Autodesk Inventor part; units mm, degrees
(part 2 of 3)
  line L709 (86.8713, 6.9678) -> (87.2019, 6.7467) construction
  line L710 (87.2019, 6.7467) -> (87.5411, 6.5326) construction
  line L711 (87.5411, 6.5326) -> (87.8883, 6.3253) construction
  line L712 (87.8883, 6.3253) -> (88.2432, 6.1246) construction
  line L713 (88.2432, 6.1246) -> (88.6055, 5.9303) construction
  line L714 (88.6055, 5.9303) -> (88.9749, 5.7423) construction
  line L715 (88.9749, 5.7423) -> (89.3511, 5.5606) construction
  line L716 (89.3511, 5.5606) -> (89.7339, 5.3851) construction
  line L717 (89.7339, 5.3851) -> (90.1231, 5.2157) construction
  line L718 (90.1231, 5.2157) -> (90.5185, 5.0524) construction
  line L719 (90.5185, 5.0524) -> (90.92, 4.8952) construction
  line L720 (90.92, 4.8952) -> (91.3274, 4.7441) construction
  line L721 (91.3274, 4.7441) -> (91.7405, 4.599) construction
  line L722 (91.7405, 4.599) -> (92.1592, 4.46) construction
  line L723 (92.1592, 4.46) -> (92.4356, 4.6954) construction
  line L724 (92.4356, 4.6954) -> (92.7102, 4.9328) construction
  line L725 (92.7102, 4.9328) -> (92.9832, 5.1722) construction
  line L726 (92.9832, 5.1722) -> (93.2544, 5.4136) construction
  line L727 (93.2544, 5.4136) -> (93.5238, 5.657) construction
  line L728 (93.5238, 5.657) -> (93.7914, 5.9023) construction
  line L729 (93.7914, 5.9023) -> (94.0572, 6.1495) construction
  line L730 (94.0572, 6.1495) -> (94.3213, 6.3987) construction
  line L731 (94.3213, 6.3987) -> (94.5835, 6.6498) construction
  line L732 (94.5835, 6.6498) -> (94.8439, 6.9028) construction
  line L733 (94.8439, 6.9028) -> (94.7449, 7.3328) construction
  line L734 (94.7449, 7.3328) -> (94.6393, 7.7577) construction
  line L735 (94.6393, 7.7577) -> (94.5272, 8.1775) construction
  line L736 (94.5272, 8.1775) -> (94.4085, 8.592) construction
  line L737 (94.4085, 8.592) -> (94.2832, 9.001) construction
  line L738 (94.2832, 9.001) -> (94.1512, 9.4044) construction
  line L739 (94.1512, 9.4044) -> (94.0125, 9.8021) construction
  line L740 (94.0125, 9.8021) -> (93.867, 10.1937) construction
  line L741 (93.867, 10.1937) -> (93.7146, 10.5791) construction
  line L742 (93.7146, 10.5791) -> (93.5553, 10.9581) construction
  line L743 (93.5553, 10.9581) -> (93.3889, 11.3303) construction
  line L744 (93.3889, 11.3303) -> (93.2152, 11.6955) construction
  line L745 (93.2152, 11.6955) -> (93.034, 12.0533) construction
  line L746 (93.034, 12.0533) -> (92.845, 12.4033) construction
  line L747 (92.845, 12.4033) -> (92.6478, 12.7449) construction
  line L748 (92.6478, 12.7449) -> (92.442, 13.0774) construction
  line L749 (92.442, 13.0774) -> (92.2268, 13.3998) construction
  line L750 (92.2268, 13.3998) -> (92.001, 13.7108) construction
  line L751 (92.001, 13.7108) -> (91.7626, 14.008) construction
  line L752 (91.7626, 14.008) -> (91.5055, 14.2844) construction
  line L753 (91.5055, 14.2844) -> (91.4052, 14.3817) construction
  line L754 (91.4052, 14.3817) -> (88.6168, 16.8782) construction
  arc A46 (88.1374, 17.5249) -> (88.6168, 16.8782) centre (89.9509, 18.3683) ccw construction
  line L755 (88.1374, 17.5249) -> (73.8914, 48.1593) construction
  line L756 (73.8914, 48.1593) -> (60.7972, 80.3007) construction
  arc A47 (60.6816, 80.6977) -> (60.7972, 80.3007) centre (62.6494, 81.0553) ccw construction
  line L757 (60.6816, 80.6977) -> (53.4682, 120.3931) construction
  circle A48 centre (-1.8122, 42.5) radius 4 construction
  line L758 (-3.103, 31.8278) -> (-3.0572, 31.8223) construction
  line L759 (-3.0572, 31.8223) -> (-3.0114, 31.8171) construction
  line L760 (-3.0114, 31.8171) -> (-2.9655, 31.8121) construction
  line L761 (-2.9655, 31.8121) -> (-2.9197, 31.8072) construction
  line L762 (-2.9197, 31.8072) -> (-2.8738, 31.8026) construction
  line L763 (-2.8738, 31.8026) -> (-2.5758, 31.7487) construction
  line L764 (-2.5758, 31.7487) -> (-2.3607, 31.6779) construction
  line L765 (-2.3607, 31.6779) -> (-2.1282, 31.5901) construction
  line L766 (-2.1282, 31.5901) -> (-1.9375, 31.49) construction
  line L767 (-1.9375, 31.49) -> (-1.7706, 31.3775) construction
  line L768 (-1.7706, 31.3775) -> (-1.6217, 31.2529) construction
  line L769 (-1.6217, 31.2529) -> (-1.477, 31.1167) construction
  line L770 (-1.477, 31.1167) -> (-1.3373, 30.9695) construction
  line L771 (-1.3373, 30.9695) -> (-1.2159, 30.8111) construction
  line L772 (-1.2159, 30.8111) -> (-1.1122, 30.6413) construction
  line L773 (-1.1122, 30.6413) -> (-1.013, 30.4611) construction
  line L774 (-1.013, 30.4611) -> (-0.9213, 30.2706) construction
  line L775 (-0.9213, 30.2706) -> (-0.8507, 30.0687) construction
  line L776 (-0.8507, 30.0687) -> (-0.7921, 29.8564) construction
  line L777 (-0.7921, 29.8564) -> (-0.7363, 29.6344) construction
  line L778 (-0.7363, 29.6344) -> (-0.7072, 29.401) construction
  line L779 (-0.7072, 29.401) -> (-0.6823, 29.1582) construction
  line L780 (-0.6823, 29.1582) -> (-0.6727, 28.9053) construction
  line L781 (-0.6727, 28.9053) -> (-0.6907, 28.6416) construction
  line L782 (-0.6907, 28.6416) -> (-0.701, 28.3702) construction
  line L783 (-0.701, 28.3702) -> (-0.5986, 27.9953) construction
  line L784 (-0.5986, 27.9953) -> (-0.4487, 27.625) construction
  line L785 (-0.4487, 27.625) -> (-0.2641, 27.2592) construction
  line L786 (-0.2641, 27.2592) -> (-0.0491, 26.8981) construction
  line L787 (-0.0491, 26.8981) -> (0.1935, 26.5424) construction
  line L788 (0.1935, 26.5424) -> (0.4621, 26.1928) construction
  line L789 (0.4621, 26.1928) -> (0.7554, 25.8498) construction
  line L790 (0.7554, 25.8498) -> (1.0724, 25.5143) construction
  line L791 (1.0724, 25.5143) -> (1.4124, 25.1869) construction
  line L792 (1.4124, 25.1869) -> (1.7746, 24.8683) construction
  line L793 (1.7746, 24.8683) -> (2.1584, 24.5594) construction
  line L794 (2.1584, 24.5594) -> (2.5632, 24.2608) construction
  line L795 (2.5632, 24.2608) -> (2.9885, 23.9733) construction
  line L796 (2.9885, 23.9733) -> (3.4338, 23.6976) construction
  line L797 (3.4338, 23.6976) -> (3.8985, 23.4344) construction
  line L798 (3.8985, 23.4344) -> (4.3822, 23.1845) construction
  line L799 (4.3822, 23.1845) -> (4.8844, 22.9487) construction
  line L800 (4.8844, 22.9487) -> (5.4044, 22.7275) construction
  line L801 (5.4044, 22.7275) -> (5.9419, 22.5218) construction
  line L802 (5.9419, 22.5218) -> (6.4962, 22.3322) construction
  line L803 (6.4962, 22.3322) -> (6.5464, 22.3529) construction
  line L804 (6.5464, 22.3529) -> (6.5966, 22.3738) construction
  line L805 (6.5966, 22.3738) -> (6.6467, 22.3948) construction
  line L806 (6.6467, 22.3948) -> (6.6967, 22.4159) construction
  line L807 (6.6967, 22.4159) -> (6.7467, 22.4372) construction
  line L808 (6.7467, 22.4372) -> (6.7967, 22.4586) construction
  line L809 (6.7967, 22.4586) -> (6.8466, 22.4801) construction
  line L810 (6.8466, 22.4801) -> (6.8964, 22.5017) construction
  line L811 (6.8964, 22.5017) -> (6.9462, 22.5235) construction
  line L812 (6.9462, 22.5235) -> (6.996, 22.5454) construction
  line L813 (6.996, 22.5454) -> (7.2427, 23.0767) construction
  line L814 (7.2427, 23.0767) -> (7.4661, 23.607) construction
  line L815 (7.4661, 23.607) -> (7.6664, 24.1355) construction
  line L816 (7.6664, 24.1355) -> (7.8437, 24.6612) construction
  line L817 (7.8437, 24.6612) -> (7.998, 25.1833) construction
  line L818 (7.998, 25.1833) -> (8.1297, 25.7009) construction
  line L819 (8.1297, 25.7009) -> (8.2389, 26.2131) construction
  line L820 (8.2389, 26.2131) -> (8.3257, 26.7191) construction
  line L821 (8.3257, 26.7191) -> (8.3903, 27.218) construction
  line L822 (8.3903, 27.218) -> (8.4329, 27.7088) construction
  line L823 (8.4329, 27.7088) -> (8.4536, 28.1907) construction
  line L824 (8.4536, 28.1907) -> (8.4525, 28.6627) construction
  line L825 (8.4525, 28.6627) -> (8.4297, 29.1237) construction
  line L826 (8.4297, 29.1237) -> (8.3851, 29.5728) construction
  line L827 (8.3851, 29.5728) -> (8.3186, 30.0087) construction
  line L828 (8.3186, 30.0087) -> (8.2298, 30.43) construction
  line L829 (8.2298, 30.43) -> (8.1179, 30.835) construction
  line L830 (8.1179, 30.835) -> (7.9816, 31.2215) construction
  line L831 (7.9816, 31.2215) -> (7.818, 31.5859) construction
  line L832 (7.818, 31.5859) -> (7.6183, 31.9192) construction
  line L833 (7.6183, 31.9192) -> (7.4153, 32.0996) construction
  line L834 (7.4153, 32.0996) -> (7.2125, 32.2692) construction
  line L835 (7.2125, 32.2692) -> (7.0366, 32.4511) construction
  line L836 (7.0366, 32.4511) -> (6.8786, 32.6371) construction
  line L837 (6.8786, 32.6371) -> (6.7302, 32.8196) construction
  line L838 (6.7302, 32.8196) -> (6.6086, 33.0136) construction
  line L839 (6.6086, 33.0136) -> (6.4959, 33.2028) construction
  line L840 (6.4959, 33.2028) -> (6.399, 33.3935) construction
  line L841 (6.399, 33.3935) -> (6.3249, 33.5916) construction
  line L842 (6.3249, 33.5916) -> (6.2635, 33.7878) construction
  line L843 (6.2635, 33.7878) -> (6.2127, 33.9802) construction
  line L844 (6.2127, 33.9802) -> (6.1824, 34.1775) construction
  line L845 (6.1824, 34.1775) -> (6.1728, 34.3802) construction
  line L846 (6.1728, 34.3802) -> (6.1746, 34.5788) construction
  line L847 (6.1746, 34.5788) -> (6.1877, 34.7726) construction
  line L848 (6.1877, 34.7726) -> (6.2221, 34.971) construction
  line L849 (6.2221, 34.971) -> (6.2818, 35.1778) construction
  line L850 (6.2818, 35.1778) -> (6.3793, 35.4064) construction
  line L851 (6.3793, 35.4064) -> (6.477, 35.6107) construction
  line L852 (6.477, 35.6107) -> (6.6444, 35.8631) construction
  line L853 (6.6444, 35.8631) -> (6.6728, 35.8994) construction
  line L854 (6.6728, 35.8994) -> (6.701, 35.9359) construction
  line L855 (6.701, 35.9359) -> (6.7291, 35.9725) construction
  line L856 (6.7291, 35.9725) -> (6.7571, 36.0092) construction
  line L857 (6.7571, 36.0092) -> (6.7848, 36.046) construction
  line L858 (6.7848, 36.046) -> (6.8124, 36.0829) construction
  line L859 (6.8124, 36.0829) -> (6.8399, 36.12) construction
  line L860 (6.8399, 36.12) -> (6.8672, 36.1572) construction
  line L861 (6.8672, 36.1572) -> (6.8943, 36.1945) construction
  line L862 (6.8943, 36.1945) -> (6.9213, 36.2319) construction
  line L863 (6.9213, 36.2319) -> (7.1169, 36.4631) construction
  line L864 (7.1169, 36.4631) -> (7.2858, 36.6139) construction
  line L865 (7.2858, 36.6139) -> (7.4781, 36.7713) construction
  line L866 (7.4781, 36.7713) -> (7.6601, 36.8864) construction
  line L867 (7.6601, 36.8864) -> (7.841, 36.9748) construction
  line L868 (7.841, 36.9748) -> (8.0234, 37.0414) construction
  line L869 (8.0234, 37.0414) -> (8.2136, 37.0986) construction
  line L870 (8.2136, 37.0986) -> (8.4109, 37.146) construction
  line L871 (8.4109, 37.146) -> (8.6089, 37.1719) construction
  line L872 (8.6089, 37.1719) -> (8.8077, 37.1769) construction
  line L873 (8.8077, 37.1769) -> (9.0134, 37.1726) construction
  line L874 (9.0134, 37.1726) -> (9.2243, 37.1568) construction
  line L875 (9.2243, 37.1568) -> (9.4344, 37.117) construction
  line L876 (9.4344, 37.117) -> (9.6476, 37.0616) construction
  line L877 (9.6476, 37.0616) -> (9.8677, 36.9989) construction
  line L878 (9.8677, 36.9989) -> (10.0844, 36.9074) construction
  line L879 (10.0844, 36.9074) -> (10.3071, 36.8076) construction
  line L880 (10.3071, 36.8076) -> (10.5309, 36.6895) construction
  line L881 (10.5309, 36.6895) -> (10.7503, 36.5421) construction
  line L882 (10.7503, 36.5421) -> (10.9802, 36.3974) construction
  line L883 (10.9802, 36.3974) -> (11.3561, 36.2987) construction
  line L884 (11.3561, 36.2987) -> (11.7516, 36.2433) construction
  line L885 (11.7516, 36.2433) -> (12.1608, 36.2203) construction
  line L886 (12.1608, 36.2203) -> (12.581, 36.2259) construction
  line L887 (12.581, 36.2259) -> (13.0103, 36.2582) construction
  line L888 (13.0103, 36.2582) -> (13.4474, 36.316) construction
  line L889 (13.4474, 36.316) -> (13.8911, 36.3985) construction
  line L890 (13.8911, 36.3985) -> (14.3402, 36.5053) construction
  line L891 (14.3402, 36.5053) -> (14.7937, 36.636) construction
  line L892 (14.7937, 36.636) -> (15.2507, 36.7904) construction
  line L893 (15.2507, 36.7904) -> (15.7101, 36.9683) construction
  line L894 (15.7101, 36.9683) -> (16.1711, 37.1696) construction
  line L895 (16.1711, 37.1696) -> (16.6328, 37.3941) construction
  line L896 (16.6328, 37.3941) -> (17.0942, 37.6419) construction
  line L897 (17.0942, 37.6419) -> (17.5545, 37.9128) construction
  line L898 (17.5545, 37.9128) -> (18.0127, 38.2068) construction
  line L899 (18.0127, 38.2068) -> (18.4681, 38.5237) construction
  line L900 (18.4681, 38.5237) -> (18.9196, 38.8635) construction
  line L901 (18.9196, 38.8635) -> (19.3665, 39.2261) construction
  line L902 (19.3665, 39.2261) -> (19.8079, 39.6113) construction
  line L903 (19.8079, 39.6113) -> (19.815, 39.6652) construction
  line L904 (19.815, 39.6652) -> (19.822, 39.7191) construction
  line L905 (19.822, 39.7191) -> (19.8289, 39.773) construction
  line L906 (19.8289, 39.773) -> (19.8356, 39.8269) construction
  line L907 (19.8356, 39.8269) -> (19.8422, 39.8808) construction
  line L908 (19.8422, 39.8808) -> (19.8486, 39.9348) construction
  line L909 (19.8486, 39.9348) -> (19.855, 39.9888) construction
  line L910 (19.855, 39.9888) -> (19.8611, 40.0427) construction
  line L911 (19.8611, 40.0427) -> (19.8672, 40.0967) construction
  line L912 (19.8672, 40.0967) -> (19.8731, 40.1508) construction
  line L913 (19.8731, 40.1508) -> (19.5363, 40.6301) construction
  line L914 (19.5363, 40.6301) -> (19.1888, 41.0888) construction
  line L915 (19.1888, 41.0888) -> (18.8312, 41.5264) construction
  line L916 (18.8312, 41.5264) -> (18.4646, 41.9428) construction
  line L917 (18.4646, 41.9428) -> (18.0897, 42.3375) construction
  line L918 (18.0897, 42.3375) -> (17.7072, 42.7104) construction
  line L919 (17.7072, 42.7104) -> (17.3182, 43.061) construction
  line L920 (17.3182, 43.061) -> (16.9234, 43.3892) construction
  line L921 (16.9234, 43.3892) -> (16.5237, 43.6946) construction
  line L922 (16.5237, 43.6946) -> (16.1199, 43.9769) construction
  line L923 (16.1199, 43.9769) -> (15.713, 44.2358) construction
  line L924 (15.713, 44.2358) -> (15.3037, 44.4708) construction
  line L925 (15.3037, 44.4708) -> (14.893, 44.6816) construction
  line L926 (14.893, 44.6816) -> (14.4818, 44.8675) construction
  line L927 (14.4818, 44.8675) -> (14.0711, 45.0279) construction
  line L928 (14.0711, 45.0279) -> (13.6618, 45.1616) construction
  line L929 (13.6618, 45.1616) -> (13.2551, 45.2672) construction
  line L930 (13.2551, 45.2672) -> (12.8522, 45.3424) construction
  line L931 (12.8522, 45.3424) -> (12.4548, 45.383) construction
  line L932 (12.4548, 45.383) -> (12.0663, 45.3767) construction
  line L933 (12.0663, 45.3767) -> (11.8085, 45.291) construction
  line L934 (11.8085, 45.291) -> (11.5603, 45.2002) construction
  line L935 (11.5603, 45.2002) -> (11.3148, 45.1388) construction
  line L936 (11.3148, 45.1388) -> (11.0747, 45.095) construction
  line L937 (11.0747, 45.095) -> (10.8425, 45.0578) construction
  line L938 (10.8425, 45.0578) -> (10.6137, 45.0494) construction
  line L939 (10.6137, 45.0494) -> (10.3934, 45.0464) construction
  line L940 (10.3934, 45.0464) -> (10.1799, 45.0579) construction
  line L941 (10.1799, 45.0579) -> (9.9713, 45.0927) construction
  line L942 (9.9713, 45.0927) -> (9.7706, 45.1376) construction
  line L943 (9.7706, 45.1376) -> (9.5787, 45.1899) construction
  line L944 (9.5787, 45.1899) -> (9.3926, 45.2622) construction
  line L945 (9.3926, 45.2622) -> (9.2123, 45.3553) construction
  line L946 (9.2123, 45.3553) -> (9.0412, 45.4562) construction
  line L947 (9.0412, 45.4562) -> (8.8799, 45.5644) construction
  line L948 (8.8799, 45.5644) -> (8.7253, 45.6933) construction
  line L949 (8.7253, 45.6933) -> (8.576, 45.8485) construction
  line L950 (8.576, 45.8485) -> (8.4268, 46.0472) construction
  line L951 (8.4268, 46.0472) -> (8.2987, 46.234) construction
  line L952 (8.2987, 46.234) -> (8.1639, 46.5051) construction
  line L953 (8.1639, 46.5051) -> (8.1466, 46.5479) construction
  line L954 (8.1466, 46.5479) -> (8.1291, 46.5906) construction
  line L955 (8.1291, 46.5906) -> (8.1115, 46.6332) construction
  line L956 (8.1115, 46.6332) -> (8.0937, 46.6758) construction
  line L957 (8.0937, 46.6758) -> (8.0757, 46.7182) construction
  line L958 (8.0757, 46.7182) -> (8.0575, 46.7606) construction
  line L959 (8.0575, 46.7606) -> (8.0391, 46.8029) construction
  line L960 (8.0391, 46.8029) -> (8.0206, 46.8451) construction
  line L961 (8.0206, 46.8451) -> (8.0018, 46.8873) construction
  line L962 (8.0018, 46.8873) -> (7.9829, 46.9293) construction
  line L963 (7.9829, 46.9293) -> (7.8805, 47.2144) construction
  line L964 (7.8805, 47.2144) -> (7.8343, 47.436) construction
  line L965 (7.8343, 47.436) -> (7.7941, 47.6813) construction
  line L966 (7.7941, 47.6813) -> (7.7854, 47.8964) construction
  line L967 (7.7854, 47.8964) -> (7.7994, 48.0973) construction
  line L968 (7.7994, 48.0973) -> (7.8329, 48.2885) construction
  line L969 (7.8329, 48.2885) -> (7.8785, 48.4819) construction
  line L970 (7.8785, 48.4819) -> (7.9361, 48.6765) construction
  line L971 (7.9361, 48.6765) -> (8.0126, 48.8608) construction
  line L972 (8.0126, 48.8608) -> (8.1077, 49.0356) construction
  line L973 (8.1077, 49.0356) -> (8.2142, 49.2115) construction
  line L974 (8.2142, 49.2115) -> (8.3334, 49.3862) construction
  line L975 (8.3334, 49.3862) -> (8.4729, 49.5483) construction
  line L976 (8.4729, 49.5483) -> (8.6275, 49.7052) construction
  line L977 (8.6275, 49.7052) -> (8.7919, 49.8645) construction
  line L978 (8.7919, 49.8645) -> (8.9794, 50.0065) construction
  line L979 (8.9794, 50.0065) -> (9.1773, 50.1494) construction
  line L980 (9.1773, 50.1494) -> (9.3914, 50.2841) construction
  line L981 (9.3914, 50.2841) -> (9.6288, 50.4005) construction
  line L982 (9.6288, 50.4005) -> (9.869, 50.5272) construction
  line L983 (9.869, 50.5272) -> (10.1425, 50.8034) construction
  line L984 (10.1425, 50.8034) -> (10.3882, 51.1183) construction
  line L985 (10.3882, 51.1183) -> (10.6127, 51.4611) construction
  line L986 (10.6127, 51.4611) -> (10.8179, 51.8278) construction
  line L987 (10.8179, 51.8278) -> (11.0047, 52.2158) construction
  line L988 (11.0047, 52.2158) -> (11.1732, 52.6232) construction
  line L989 (11.1732, 52.6232) -> (11.3235, 53.0487) construction
  line L990 (11.3235, 53.0487) -> (11.4556, 53.491) construction
  line L991 (11.4556, 53.491) -> (11.5692, 53.9491) construction
  line L992 (11.5692, 53.9491) -> (11.6639, 54.4221) construction
  line L993 (11.6639, 54.4221) -> (11.7396, 54.9089) construction
  line L994 (11.7396, 54.9089) -> (11.7958, 55.4088) construction
  line L995 (11.7958, 55.4088) -> (11.8321, 55.9209) construction
  line L996 (11.8321, 55.9209) -> (11.8483, 56.4444) construction
  line L997 (11.8483, 56.4444) -> (11.8438, 56.9784) construction
  line L998 (11.8438, 56.9784) -> (11.8183, 57.5223) construction
  line L999 (11.8183, 57.5223) -> (11.7715, 58.0751) construction
  line L1000 (11.7715, 58.0751) -> (11.703, 58.636) construction
  line L1001 (11.703, 58.636) -> (11.6125, 59.2043) construction
  line L1002 (11.6125, 59.2043) -> (11.4995, 59.7792) construction
  line L1003 (11.4995, 59.7792) -> (11.4564, 59.8123) construction
  line L1004 (11.4564, 59.8123) -> (11.4133, 59.8453) construction
  line L1005 (11.4133, 59.8453) -> (11.37, 59.8782) construction
  line L1006 (11.37, 59.8782) -> (11.3267, 59.911) construction
  line L1007 (11.3267, 59.911) -> (11.2833, 59.9436) construction
  line L1008 (11.2833, 59.9436) -> (11.2398, 59.9762) construction
  line L1009 (11.2398, 59.9762) -> (11.1962, 60.0087) construction
  line L1010 (11.1962, 60.0087) -> (11.1525, 60.041) construction
  line L1011 (11.1525, 60.041) -> (11.1088, 60.0733) construction
  line L1012 (11.1088, 60.0733) -> (11.065, 60.1054) construction
  line L1013 (11.065, 60.1054) -> (10.4815, 60.0534) construction
  line L1014 (10.4815, 60.0534) -> (9.9105, 59.9817) construction
  line L1015 (9.9105, 59.9817) -> (9.3527, 59.8909) construction
  line L1016 (9.3527, 59.8909) -> (8.8088, 59.7816) construction
  line L1017 (8.8088, 59.7816) -> (8.2794, 59.6543) construction
  line L1018 (8.2794, 59.6543) -> (7.7654, 59.5095) construction
  line L1019 (7.7654, 59.5095) -> (7.2672, 59.3479) construction
  line L1020 (7.2672, 59.3479) -> (6.7856, 59.1701) construction
  line L1021 (6.7856, 59.1701) -> (6.3212, 58.9766) construction
  line L1022 (6.3212, 58.9766) -> (5.8749, 58.7681) construction
  line L1023 (5.8749, 58.7681) -> (5.4472, 58.5451) construction
  line L1024 (5.4472, 58.5451) -> (5.039, 58.3082) construction
  line L1025 (5.039, 58.3082) -> (4.6511, 58.0579) construction
  line L1026 (4.6511, 58.0579) -> (4.2845, 57.7947) construction
  line L1027 (4.2845, 57.7947) -> (3.9403, 57.5192) construction
  line L1028 (3.9403, 57.5192) -> (3.6198, 57.2316) construction
  line L1029 (3.6198, 57.2316) -> (3.325, 56.9322) construction
  line L1030 (3.325, 56.9322) -> (3.0584, 56.6209) construction
  line L1031 (3.0584, 56.6209) -> (2.8246, 56.2971) construction
  line L1032 (2.8246, 56.2971) -> (2.6358, 55.9574) construction
  line L1033 (2.6358, 55.9574) -> (2.5811, 55.6914) construction
  line L1034 (2.5811, 55.6914) -> (2.5357, 55.431) construction
  line L1035 (2.5357, 55.431) -> (2.466, 55.1877) construction
  line L1036 (2.466, 55.1877) -> (2.384, 54.9579) construction
  line L1037 (2.384, 54.9579) -> (2.3001, 54.7381) construction
  line L1038 (2.3001, 54.7381) -> (2.193, 54.5358) construction
  line L1039 (2.193, 54.5358) -> (2.0854, 54.3436) construction
  line L1040 (2.0854, 54.3436) -> (1.9687, 54.1644) construction
  line L1041 (1.9687, 54.1644) -> (1.8342, 54.0012) construction
  line L1042 (1.8342, 54.0012) -> (1.695, 53.8498) construction
  line L1043 (1.695, 53.8498) -> (1.5537, 53.7097) construction
  line L1044 (1.5537, 53.7097) -> (1.3981, 53.5847) construction
  line L1045 (1.3981, 53.5847) -> (1.2273, 53.4751) construction
  line L1046 (1.2273, 53.4751) -> (1.0544, 53.3774) construction
  line L1047 (1.0544, 53.3774) -> (0.88, 53.2918) construction
  line L1048 (0.88, 53.2918) -> (0.6911, 53.2224) construction
  line L1049 (0.6911, 53.2224) -> (0.482, 53.1707) construction
  line L1050 (0.482, 53.1707) -> (0.2353, 53.1408) construction
  line L1051 (0.2353, 53.1408) -> (0.0096, 53.1233) construction
  line L1052 (0.0096, 53.1233) -> (-0.2927, 53.1421) construction
  line L1053 (-0.2927, 53.1421) -> (-0.3384, 53.1485) construction
  line L1054 (-0.3384, 53.1485) -> (-0.3841, 53.1547) construction
  line L1055 (-0.3841, 53.1547) -> (-0.4298, 53.1608) construction
  line L1056 (-0.4298, 53.1608) -> (-0.4756, 53.1666) construction
  line L1057 (-0.4756, 53.1666) -> (-0.5213, 53.1722) construction
  line L1058 (-0.5213, 53.1722) -> (-0.5671, 53.1777) construction
  line L1059 (-0.5671, 53.1777) -> (-0.613, 53.1829) construction
  line L1060 (-0.613, 53.1829) -> (-0.6588, 53.188) construction
  line L1061 (-0.6588, 53.188) -> (-0.7047, 53.1928) construction
  line L1062 (-0.7047, 53.1928) -> (-0.7506, 53.1975) construction
  line L1063 (-0.7506, 53.1975) -> (-1.0486, 53.2513) construction
  line L1064 (-1.0486, 53.2513) -> (-1.2636, 53.3221) construction
  line L1065 (-1.2636, 53.3221) -> (-1.4961, 53.4099) construction
  line L1066 (-1.4961, 53.4099) -> (-1.6868, 53.51) construction
  line L1067 (-1.6868, 53.51) -> (-1.8538, 53.6225) construction
  line L1068 (-1.8538, 53.6225) -> (-2.0027, 53.7471) construction
  line L1069 (-2.0027, 53.7471) -> (-2.1473, 53.8833) construction
  line L1070 (-2.1473, 53.8833) -> (-2.2871, 54.0305) construction
  line L1071 (-2.2871, 54.0305) -> (-2.4084, 54.1889) construction
  line L1072 (-2.4084, 54.1889) -> (-2.5122, 54.3587) construction
  line L1073 (-2.5122, 54.3587) -> (-2.6113, 54.5389) construction
  line L1074 (-2.6113, 54.5389) -> (-2.703, 54.7294) construction
  line L1075 (-2.703, 54.7294) -> (-2.7736, 54.9313) construction
  line L1076 (-2.7736, 54.9313) -> (-2.8322, 55.1437) construction
  line L1077 (-2.8322, 55.1437) -> (-2.888, 55.3656) construction
  line L1078 (-2.888, 55.3656) -> (-2.9171, 55.599) construction
  line L1079 (-2.9171, 55.599) -> (-2.942, 55.8418) construction
  line L1080 (-2.942, 55.8418) -> (-2.9516, 56.0947) construction
  line L1081 (-2.9516, 56.0947) -> (-2.9337, 56.3584) construction
  line L1082 (-2.9337, 56.3584) -> (-2.9234, 56.6298) construction
  line L1083 (-2.9234, 56.6298) -> (-3.0258, 57.0047) construction
  line L1084 (-3.0258, 57.0047) -> (-3.1756, 57.375) construction
  line L1085 (-3.1756, 57.375) -> (-3.3603, 57.7408) construction
  line L1086 (-3.3603, 57.7408) -> (-3.5752, 58.1019) construction
  line L1087 (-3.5752, 58.1019) -> (-3.8179, 58.4576) construction
  line L1088 (-3.8179, 58.4576) -> (-4.0865, 58.8072) construction
  line L1089 (-4.0865, 58.8072) -> (-4.3798, 59.1502) construction
  line L1090 (-4.3798, 59.1502) -> (-4.6968, 59.4857) construction
  line L1091 (-4.6968, 59.4857) -> (-5.0367, 59.8132) construction
  line L1092 (-5.0367, 59.8132) -> (-5.3989, 60.1317) construction
  line L1093 (-5.3989, 60.1317) -> (-5.7827, 60.4406) construction
  line L1094 (-5.7827, 60.4406) -> (-6.1875, 60.7392) construction
  line L1095 (-6.1875, 60.7392) -> (-6.6128, 61.0268) construction
  line L1096 (-6.6128, 61.0268) -> (-7.0581, 61.3025) construction
  line L1097 (-7.0581, 61.3025) -> (-7.5229, 61.5656) construction
  line L1098 (-7.5229, 61.5656) -> (-8.0066, 61.8155) construction
  line L1099 (-8.0066, 61.8155) -> (-8.5087, 62.0513) construction
  line L1100 (-8.5087, 62.0513) -> (-9.0288, 62.2725) construction
  line L1101 (-9.0288, 62.2725) -> (-9.5662, 62.4782) construction
  line L1102 (-9.5662, 62.4782) -> (-10.1205, 62.6679) construction
  line L1103 (-10.1205, 62.6679) -> (-10.1707, 62.6471) construction
  line L1104 (-10.1707, 62.6471) -> (-10.2209, 62.6262) construction
  line L1105 (-10.2209, 62.6262) -> (-10.271, 62.6052) construction
  line L1106 (-10.271, 62.6052) -> (-10.3211, 62.5841) construction
  line L1107 (-10.3211, 62.5841) -> (-10.3711, 62.5628) construction
  line L1108 (-10.3711, 62.5628) -> (-10.421, 62.5414) construction
  line L1109 (-10.421, 62.5414) -> (-10.4709, 62.5199) construction
  line L1110 (-10.4709, 62.5199) -> (-10.5208, 62.4983) construction
  line L1111 (-10.5208, 62.4983) -> (-10.5706, 62.4765) construction
  line L1112 (-10.5706, 62.4765) -> (-10.6203, 62.4546) construction
  line L1113 (-10.6203, 62.4546) -> (-10.867, 61.9233) construction
  line L1114 (-10.867, 61.9233) -> (-11.0905, 61.393) construction
  line L1115 (-11.0905, 61.393) -> (-11.2907, 60.8645) construction
  line L1116 (-11.2907, 60.8645) -> (-11.468, 60.3388) construction
  line L1117 (-11.468, 60.3388) -> (-11.6224, 59.8167) construction
  line L1118 (-11.6224, 59.8167) -> (-11.7541, 59.2991) construction
  line L1119 (-11.7541, 59.2991) -> (-11.8632, 58.7869) construction
  line L1120 (-11.8632, 58.7869) -> (-11.95, 58.2809) construction
  line L1121 (-11.95, 58.2809) -> (-12.0146, 57.7821) construction
  line L1122 (-12.0146, 57.7821) -> (-12.0572, 57.2912) construction
  line L1123 (-12.0572, 57.2912) -> (-12.0779, 56.8093) construction
  line L1124 (-12.0779, 56.8093) -> (-12.0769, 56.3374) construction
  line L1125 (-12.0769, 56.3374) -> (-12.0541, 55.8763) construction
  line L1126 (-12.0541, 55.8763) -> (-12.0095, 55.4272) construction
  line L1127 (-12.0095, 55.4272) -> (-11.943, 54.9914) construction
  line L1128 (-11.943, 54.9914) -> (-11.8541, 54.5701) construction
  line L1129 (-11.8541, 54.5701) -> (-11.7423, 54.165) construction
  line L1130 (-11.7423, 54.165) -> (-11.606, 53.7785) construction
  line L1131 (-11.606, 53.7785) -> (-11.4424, 53.4141) construction
  line L1132 (-11.4424, 53.4141) -> (-11.2426, 53.0808) construction
  line L1133 (-11.2426, 53.0808) -> (-11.0396, 52.9004) construction
  line L1134 (-11.0396, 52.9004) -> (-10.8368, 52.7308) construction
  line L1135 (-10.8368, 52.7308) -> (-10.6609, 52.5489) construction
  line L1136 (-10.6609, 52.5489) -> (-10.5029, 52.3629) construction
  line L1137 (-10.5029, 52.3629) -> (-10.3546, 52.1804) construction
  line L1138 (-10.3546, 52.1804) -> (-10.2329, 51.9865) construction
  line L1139 (-10.2329, 51.9865) -> (-10.1202, 51.7972) construction
  line L1140 (-10.1202, 51.7972) -> (-10.0234, 51.6065) construction
  line L1141 (-10.0234, 51.6065) -> (-9.9493, 51.4084) construction
  line L1142 (-9.9493, 51.4084) -> (-9.8878, 51.2122) construction
  line L1143 (-9.8878, 51.2122) -> (-9.8371, 51.0198) construction
  line L1144 (-9.8371, 51.0198) -> (-9.8067, 50.8226) construction
  line L1145 (-9.8067, 50.8226) -> (-9.7972, 50.6198) construction
  line L1146 (-9.7972, 50.6198) -> (-9.799, 50.4212) construction
  line L1147 (-9.799, 50.4212) -> (-9.812, 50.2274) construction
  line L1148 (-9.812, 50.2274) -> (-9.8464, 50.029) construction
  line L1149 (-9.8464, 50.029) -> (-9.9061, 49.8222) construction
  line L1150 (-9.9061, 49.8222) -> (-10.0036, 49.5936) construction
  line L1151 (-10.0036, 49.5936) -> (-10.1013, 49.3893) construction
  line L1152 (-10.1013, 49.3893) -> (-10.2687, 49.1369) construction
  line L1153 (-10.2687, 49.1369) -> (-10.2971, 49.1006) construction
  line L1154 (-10.2971, 49.1006) -> (-10.3254, 49.0641) construction
  line L1155 (-10.3254, 49.0641) -> (-10.3535, 49.0275) construction
  line L1156 (-10.3535, 49.0275) -> (-10.3814, 48.9908) construction
  line L1157 (-10.3814, 48.9908) -> (-10.4092, 48.954) construction
  line L1158 (-10.4092, 48.954) -> (-10.4368, 48.9171) construction
  line L1159 (-10.4368, 48.9171) -> (-10.4642, 48.88) construction
  line L1160 (-10.4642, 48.88) -> (-10.4915, 48.8428) construction
  line L1161 (-10.4915, 48.8428) -> (-10.5187, 48.8055) construction
  line L1162 (-10.5187, 48.8055) -> (-10.5456, 48.7681) construction
  line L1163 (-10.5456, 48.7681) -> (-10.7413, 48.5369) construction
  line L1164 (-10.7413, 48.5369) -> (-10.9101, 48.3861) construction
  line L1165 (-10.9101, 48.3861) -> (-11.1024, 48.2287) construction
  line L1166 (-11.1024, 48.2287) -> (-11.2844, 48.1136) construction
  line L1167 (-11.2844, 48.1136) -> (-11.4653, 48.0252) construction
  line L1168 (-11.4653, 48.0252) -> (-11.6477, 47.9586) construction
  line L1169 (-11.6477, 47.9586) -> (-11.838, 47.9014) construction
  line L1170 (-11.838, 47.9014) -> (-12.0353, 47.854) construction
  line L1171 (-12.0353, 47.854) -> (-12.2332, 47.8281) construction
  line L1172 (-12.2332, 47.8281) -> (-12.4321, 47.8231) construction
  line L1173 (-12.4321, 47.8231) -> (-12.6377, 47.8274) construction
  line L1174 (-12.6377, 47.8274) -> (-12.8486, 47.8432) construction
  line L1175 (-12.8486, 47.8432) -> (-13.0587, 47.883) construction
  line L1176 (-13.0587, 47.883) -> (-13.2719, 47.9384) construction
  line L1177 (-13.2719, 47.9384) -> (-13.4921, 48.0011) construction
  line L1178 (-13.4921, 48.0011) -> (-13.7088, 48.0926) construction
  line L1179 (-13.7088, 48.0926) -> (-13.9314, 48.1924) construction
  line L1180 (-13.9314, 48.1924) -> (-14.1552, 48.3105) construction
  line L1181 (-14.1552, 48.3105) -> (-14.3746, 48.4579) construction
  line L1182 (-14.3746, 48.4579) -> (-14.6046, 48.6026) construction
  line L1183 (-14.6046, 48.6026) -> (-14.9804, 48.7013) construction
  line L1184 (-14.9804, 48.7013) -> (-15.376, 48.7567) construction
  line L1185 (-15.376, 48.7567) -> (-15.7852, 48.7797) construction
  line L1186 (-15.7852, 48.7797) -> (-16.2053, 48.7741) construction
  line L1187 (-16.2053, 48.7741) -> (-16.6347, 48.7418) construction
  line L1188 (-16.6347, 48.7418) -> (-17.0718, 48.684) construction
  line L1189 (-17.0718, 48.684) -> (-17.5155, 48.6015) construction
  line L1190 (-17.5155, 48.6015) -> (-17.9646, 48.4947) construction
  line L1191 (-17.9646, 48.4947) -> (-18.4181, 48.364) construction
  line L1192 (-18.4181, 48.364) -> (-18.875, 48.2096) construction
  line L1193 (-18.875, 48.2096) -> (-19.3345, 48.0317) construction
  line L1194 (-19.3345, 48.0317) -> (-19.7955, 47.8305) construction
  line L1195 (-19.7955, 47.8305) -> (-20.2571, 47.6059) construction
  line L1196 (-20.2571, 47.6059) -> (-20.7185, 47.3581) construction
  line L1197 (-20.7185, 47.3581) -> (-21.1788, 47.0872) construction
  line L1198 (-21.1788, 47.0872) -> (-21.6371, 46.7932) construction
  line L1199 (-21.6371, 46.7932) -> (-22.0924, 46.4763) construction
  line L1200 (-22.0924, 46.4763) -> (-22.544, 46.1365) construction
  line L1201 (-22.544, 46.1365) -> (-22.9909, 45.7739) construction
  line L1202 (-22.9909, 45.7739) -> (-23.4322, 45.3887) construction
  line L1203 (-23.4322, 45.3887) -> (-23.4393, 45.3348) construction
  line L1204 (-23.4393, 45.3348) -> (-23.4463, 45.2809) construction
  line L1205 (-23.4463, 45.2809) -> (-23.4532, 45.227) construction
  line L1206 (-23.4532, 45.227) -> (-23.4599, 45.1731) construction
  line L1207 (-23.4599, 45.1731) -> (-23.4665, 45.1192) construction
  line L1208 (-23.4665, 45.1192) -> (-23.473, 45.0652) construction
  line L1209 (-23.473, 45.0652) -> (-23.4793, 45.0113) construction
  line L1210 (-23.4793, 45.0113) -> (-23.4855, 44.9573) construction
  line L1211 (-23.4855, 44.9573) -> (-23.4915, 44.9033) construction
  line L1212 (-23.4915, 44.9033) -> (-23.4975, 44.8492) construction
  line L1213 (-23.4975, 44.8492) -> (-23.1607, 44.3699) construction
  line L1214 (-23.1607, 44.3699) -> (-22.8131, 43.9112) construction
  line L1215 (-22.8131, 43.9112) -> (-22.4556, 43.4736) construction
  line L1216 (-22.4556, 43.4736) -> (-22.0889, 43.0572) construction
  line L1217 (-22.0889, 43.0572) -> (-21.714, 42.6625) construction
  line L1218 (-21.714, 42.6625) -> (-21.3316, 42.2896) construction
  line L1219 (-21.3316, 42.2896) -> (-20.9426, 41.939) construction
  line L1220 (-20.9426, 41.939) -> (-20.5478, 41.6108) construction
  line L1221 (-20.5478, 41.6108) -> (-20.148, 41.3054) construction
  line L1222 (-20.148, 41.3054) -> (-19.7443, 41.0231) construction
  line L1223 (-19.7443, 41.0231) -> (-19.3373, 40.7643) construction
  line L1224 (-19.3373, 40.7643) -> (-18.928, 40.5292) construction
  line L1225 (-18.928, 40.5292) -> (-18.5173, 40.3184) construction
  line L1226 (-18.5173, 40.3184) -> (-18.1061, 40.1325) construction
  line L1227 (-18.1061, 40.1325) -> (-17.6954, 39.9722) construction
  line L1228 (-17.6954, 39.9722) -> (-17.2861, 39.8384) construction
  line L1229 (-17.2861, 39.8384) -> (-16.8794, 39.7328) construction
  line L1230 (-16.8794, 39.7328) -> (-16.4766, 39.6576) construction
  line L1231 (-16.4766, 39.6576) -> (-16.0792, 39.6171) construction
  line L1232 (-16.0792, 39.6171) -> (-15.6906, 39.6234) construction
  line L1233 (-15.6906, 39.6234) -> (-15.4329, 39.709) construction
  line L1234 (-15.4329, 39.709) -> (-15.1846, 39.7999) construction
  line L1235 (-15.1846, 39.7999) -> (-14.9391, 39.8612) construction
  line L1236 (-14.9391, 39.8612) -> (-14.6991, 39.9051) construction
  line L1237 (-14.6991, 39.9051) -> (-14.4668, 39.9423) construction
  line L1238 (-14.4668, 39.9423) -> (-14.2381, 39.9506) construction
  line L1239 (-14.2381, 39.9506) -> (-14.0178, 39.9536) construction
  line L1240 (-14.0178, 39.9536) -> (-13.8043, 39.9422) construction
  line L1241 (-13.8043, 39.9422) -> (-13.5957, 39.9073) construction
  line L1242 (-13.5957, 39.9073) -> (-13.395, 39.8624) construction
  line L1243 (-13.395, 39.8624) -> (-13.203, 39.8101) construction
  line L1244 (-13.203, 39.8101) -> (-13.017, 39.7378) construction
  line L1245 (-13.017, 39.7378) -> (-12.8366, 39.6447) construction
  line L1246 (-12.8366, 39.6447) -> (-12.6655, 39.5438) construction
  line L1247 (-12.6655, 39.5438) -> (-12.5042, 39.4356) construction
  line L1248 (-12.5042, 39.4356) -> (-12.3496, 39.3067) construction
  line L1249 (-12.3496, 39.3067) -> (-12.2003, 39.1515) construction
  line L1250 (-12.2003, 39.1515) -> (-12.0511, 38.9528) construction
  line L1251 (-12.0511, 38.9528) -> (-11.9231, 38.766) construction
  line L1252 (-11.9231, 38.766) -> (-11.7882, 38.4949) construction
  line L1253 (-11.7882, 38.4949) -> (-11.7709, 38.4521) construction
  line L1254 (-11.7709, 38.4521) -> (-11.7535, 38.4094) construction
  line L1255 (-11.7535, 38.4094) -> (-11.7358, 38.3668) construction
  line L1256 (-11.7358, 38.3668) -> (-11.718, 38.3243) construction
  line L1257 (-11.718, 38.3243) -> (-11.7, 38.2818) construction
  line L1258 (-11.7, 38.2818) -> (-11.6818, 38.2394) construction
  line L1259 (-11.6818, 38.2394) -> (-11.6634, 38.1971) construction
  line L1260 (-11.6634, 38.1971) -> (-11.6449, 38.1549) construction
  line L1261 (-11.6449, 38.1549) -> (-11.6262, 38.1127) construction
  line L1262 (-11.6262, 38.1127) -> (-11.6072, 38.0707) construction
  line L1263 (-11.6072, 38.0707) -> (-11.5048, 37.7856) construction
  line L1264 (-11.5048, 37.7856) -> (-11.4586, 37.564) construction
  line L1265 (-11.4586, 37.564) -> (-11.4185, 37.3187) construction
  line L1266 (-11.4185, 37.3187) -> (-11.4098, 37.1036) construction
  line L1267 (-11.4098, 37.1036) -> (-11.4237, 36.9027) construction
  line L1268 (-11.4237, 36.9027) -> (-11.4572, 36.7115) construction
  line L1269 (-11.4572, 36.7115) -> (-11.5028, 36.5181) construction
  line L1270 (-11.5028, 36.5181) -> (-11.5604, 36.3235) construction
  line L1271 (-11.5604, 36.3235) -> (-11.637, 36.1392) construction
  line L1272 (-11.637, 36.1392) -> (-11.7321, 35.9644) construction
  line L1273 (-11.7321, 35.9644) -> (-11.8386, 35.7885) construction
  line L1274 (-11.8386, 35.7885) -> (-11.9577, 35.6138) construction
  line L1275 (-11.9577, 35.6138) -> (-12.0972, 35.4517) construction
  line L1276 (-12.0972, 35.4517) -> (-12.2519, 35.2948) construction
  line L1277 (-12.2519, 35.2948) -> (-12.4162, 35.1355) construction
  line L1278 (-12.4162, 35.1355) -> (-12.6038, 34.9936) construction
  line L1279 (-12.6038, 34.9936) -> (-12.8016, 34.8506) construction
  line L1280 (-12.8016, 34.8506) -> (-13.0158, 34.7159) construction
  line L1281 (-13.0158, 34.7159) -> (-13.2531, 34.5996) construction
  line L1282 (-13.2531, 34.5996) -> (-13.4933, 34.4728) construction
  line L1283 (-13.4933, 34.4728) -> (-13.7668, 34.1966) construction
  line L1284 (-13.7668, 34.1966) -> (-14.0125, 33.8818) construction
  line L1285 (-14.0125, 33.8818) -> (-14.2371, 33.5389) construction
  line L1286 (-14.2371, 33.5389) -> (-14.4423, 33.1722) construction
  line L1287 (-14.4423, 33.1722) -> (-14.629, 32.7842) construction
  line L1288 (-14.629, 32.7842) -> (-14.7975, 32.3768) construction
  line L1289 (-14.7975, 32.3768) -> (-14.9479, 31.9513) construction
  line L1290 (-14.9479, 31.9513) -> (-15.0799, 31.509) construction
  line L1291 (-15.0799, 31.509) -> (-15.1935, 31.0509) construction
  line L1292 (-15.1935, 31.0509) -> (-15.2883, 30.578) construction
  line L1293 (-15.2883, 30.578) -> (-15.3639, 30.0911) construction
  line L1294 (-15.3639, 30.0911) -> (-15.4201, 29.5912) construction
  line L1295 (-15.4201, 29.5912) -> (-15.4565, 29.0791) construction
  line L1296 (-15.4565, 29.0791) -> (-15.4726, 28.5557) construction
  line L1297 (-15.4726, 28.5557) -> (-15.4681, 28.0216) construction
  line L1298 (-15.4681, 28.0216) -> (-15.4427, 27.4778) construction
  line L1299 (-15.4427, 27.4778) -> (-15.3959, 26.925) construction
  line L1300 (-15.3959, 26.925) -> (-15.3273, 26.364) construction
  line L1301 (-15.3273, 26.364) -> (-15.2368, 25.7957) construction
  line L1302 (-15.2368, 25.7957) -> (-15.1239, 25.2208) construction
  line L1303 (-15.1239, 25.2208) -> (-15.0808, 25.1877) construction
  line L1304 (-15.0808, 25.1877) -> (-15.0376, 25.1547) construction
  line L1305 (-15.0376, 25.1547) -> (-14.9944, 25.1218) construction
  line L1306 (-14.9944, 25.1218) -> (-14.951, 25.0891) construction
  line L1307 (-14.951, 25.0891) -> (-14.9076, 25.0564) construction
  line L1308 (-14.9076, 25.0564) -> (-14.8641, 25.0238) construction
  line L1309 (-14.8641, 25.0238) -> (-14.8205, 24.9913) construction
  line L1310 (-14.8205, 24.9913) -> (-14.7769, 24.959) construction
  line L1311 (-14.7769, 24.959) -> (-14.7331, 24.9267) construction
  line L1312 (-14.7331, 24.9267) -> (-14.6893, 24.8946) construction
  line L1313 (-14.6893, 24.8946) -> (-14.1058, 24.9466) construction
  line L1314 (-14.1058, 24.9466) -> (-13.5348, 25.0183) construction
  line L1315 (-13.5348, 25.0183) -> (-12.977, 25.1091) construction
  line L1316 (-12.977, 25.1091) -> (-12.4331, 25.2184) construction
  line L1317 (-12.4331, 25.2184) -> (-11.9038, 25.3458) construction
  line L1318 (-11.9038, 25.3458) -> (-11.3897, 25.4905) construction
  line L1319 (-11.3897, 25.4905) -> (-10.8915, 25.6521) construction
  line L1320 (-10.8915, 25.6521) -> (-10.4099, 25.8299) construction
  line L1321 (-10.4099, 25.8299) -> (-9.9456, 26.0234) construction
  line L1322 (-9.9456, 26.0234) -> (-9.4992, 26.2319) construction
  line L1323 (-9.4992, 26.2319) -> (-9.0715, 26.4549) construction
  line L1324 (-9.0715, 26.4549) -> (-8.6633, 26.6918) construction
  line L1325 (-8.6633, 26.6918) -> (-8.2754, 26.9421) construction
  line L1326 (-8.2754, 26.9421) -> (-7.9088, 27.2053) construction
  line L1327 (-7.9088, 27.2053) -> (-7.5646, 27.4808) construction
  line L1328 (-7.5646, 27.4808) -> (-7.2442, 27.7684) construction
  line L1329 (-7.2442, 27.7684) -> (-6.9493, 28.0678) construction
  line L1330 (-6.9493, 28.0678) -> (-6.6828, 28.3791) construction
  line L1331 (-6.6828, 28.3791) -> (-6.449, 28.7029) construction
  line L1332 (-6.449, 28.7029) -> (-6.2601, 29.0426) construction
  line L1333 (-6.2601, 29.0426) -> (-6.2054, 29.3086) construction
  line L1334 (-6.2054, 29.3086) -> (-6.16, 29.569) construction
  line L1335 (-6.16, 29.569) -> (-6.0904, 29.8123) construction
  line L1336 (-6.0904, 29.8123) -> (-6.0083, 30.0422) construction
  line L1337 (-6.0083, 30.0422) -> (-5.9244, 30.2619) construction
  line L1338 (-5.9244, 30.2619) -> (-5.8173, 30.4642) construction
  line L1339 (-5.8173, 30.4642) -> (-5.7097, 30.6564) construction
  line L1340 (-5.7097, 30.6564) -> (-5.5931, 30.8356) construction
  line L1341 (-5.5931, 30.8356) -> (-5.4586, 30.9988) construction
  line L1342 (-5.4586, 30.9988) -> (-5.3193, 31.1502) construction
  line L1343 (-5.3193, 31.1502) -> (-5.1781, 31.2903) construction
  line L1344 (-5.1781, 31.2903) -> (-5.0224, 31.4153) construction
  line L1345 (-5.0224, 31.4153) -> (-4.8516, 31.5249) construction
  line L1346 (-4.8516, 31.5249) -> (-4.6787, 31.6227) construction
  line L1347 (-4.6787, 31.6227) -> (-4.5044, 31.7082) construction
  line L1348 (-4.5044, 31.7082) -> (-4.3154, 31.7776) construction
  line L1349 (-4.3154, 31.7776) -> (-4.1064, 31.8293) construction
  line L1350 (-4.1064, 31.8293) -> (-3.8597, 31.8592) construction
  line L1351 (-3.8597, 31.8592) -> (-3.6339, 31.8767) construction
  line L1352 (-3.6339, 31.8767) -> (-3.3316, 31.8579) construction
  line L1353 (-3.3316, 31.8579) -> (-3.286, 31.8515) construction
  line L1354 (-3.286, 31.8515) -> (-3.2403, 31.8453) construction
  line L1355 (-3.2403, 31.8453) -> (-3.1945, 31.8393) construction
  line L1356 (-3.1945, 31.8393) -> (-3.1488, 31.8334) construction
  line L1357 (-3.1488, 31.8334) -> (-3.103, 31.8278) construction
  arc A49 (94, 17) -> (96.3186, 21.9037) centre (94, 20) ccw
  circle A50 centre (-1.8122, 42.5) radius 22 construction
  circle A51 centre (60, 42.5) radius 50 construction
  arc A52 (9.3779, 17.4763) -> (11, 17) centre (11, 20) ccw
  circle A53 centre (11, 20) radius 1.6
  circle A54 centre (94, 20) radius 1.6
  line L1358 (180, -7.5) -> (180, 42.5)
  arc A55 (180, 42.5) -> (-60, 42.5) centre (60, 42.5) ccw
  line L1359 (-60, 42.5) -> (-60, -7.5)
  arc A56 (11.6137, 67.9366) -> (9.3779, 67.5237) centre (11, 65) ccw
  circle A57 centre (11, 65) radius 1.6
  circle A58 centre (120, 0) radius 1.6
  arc A59 (53.6424, 73.8621) -> (29.6315, 32.4127) centre (60, 42.5) ccw construction
  arc A60 (56.0387, 71.9671) -> (53.6424, 73.8621) centre (54.0397, 71.902) ccw construction
  line L1360 (56.0387, 71.9671) -> (56.4727, 58.6418) construction
  arc A61 (55.1239, 56.6853) -> (56.4727, 58.6418) centre (54.4737, 58.5767) ccw construction
  arc A62 (55.1239, 56.6853) -> (46.9019, 35.1898) centre (60, 42.5) ccw construction
  arc A63 (45.3269, 32.2224) -> (46.9019, 35.1898) centre (45.1555, 34.2151) ccw construction
  line L1361 (45.3269, 32.2224) -> (31.7009, 31.0505) construction
  arc A64 (29.6315, 32.4127) -> (31.7009, 31.0505) centre (31.5295, 33.0431) ccw construction
  arc A65 (67.4433, 55.5229) -> (63.9427, 56.9726) centre (60, 42.5) ccw construction
  arc A66 (62.4695, 58.8371) -> (63.9427, 56.9726) centre (64.4684, 58.9022) ccw construction
  line L1362 (62.4695, 58.8371) -> (62.0355, 72.1624) construction
  arc A67 (64.3034, 74.2093) -> (62.0355, 72.1624) centre (64.0344, 72.2275) ccw construction
  arc A68 (66.7389, 73.7824) -> (64.3034, 74.2093) centre (60, 42.5) ccw construction
  arc A69 (67.1587, 73.6418) -> (66.7389, 73.7824) centre (66.3177, 71.8272) ccw construction
  line L1363 (67.1587, 73.6418) -> (83.4708, 66.0814) construction
  arc A70 (83.5152, 62.4734) -> (83.4708, 66.0814) centre (82.6298, 64.2668) ccw construction
  line L1364 (83.5152, 62.4734) -> (69.3211, 55.466) construction
  arc A71 (67.4433, 55.5229) -> (69.3211, 55.466) centre (68.4358, 57.2593) ccw construction
  arc A72 (133.9483, 39.733) -> (130.0964, 66.217) centre (60, 42.5) ccw construction
  arc A73 (131.6118, 37.8365) -> (133.9483, 39.733) centre (131.9496, 39.8078) ccw construction
  line L1365 (131.6118, 37.8365) -> (90.0847, 44.9534) construction
  arc A74 (89.5372, 48.7181) -> (90.0847, 44.9534) centre (90.4226, 46.9247) ccw construction
  line L1366 (89.5372, 48.7181) -> (127.3165, 67.3694) construction
  arc A75 (130.0964, 66.217) -> (127.3165, 67.3694) centre (128.2019, 65.576) ccw construction
  circle A76 centre (60, 42.5) radius 4 construction
  circle A77 centre (103.9372, 64.1914) radius 1.2295 construction
  circle A78 centre (108.2959, 34.2231) radius 1.2295 construction
  circle A79 centre (93.5114, 36.7568) radius 1.2295 construction
  circle A80 centre (90.4871, 57.5512) radius 1.2295 construction
  arc A81 (135.4209, 21.965) -> (137.7013, 23.4603) centre (135.7588, 23.9363) ccw construction
  arc A82 (137.7013, 23.4603) -> (129.0585, 82.8846) centre (60, 42.5) ccw construction
  arc A83 (129.0585, 82.8846) -> (126.4467, 83.6684) centre (127.3321, 81.875) ccw construction
  line L1367 (126.4467, 83.6684) -> (95.0687, 68.1773) construction
  arc A84 (93.2799, 68.1863) -> (95.0687, 68.1773) centre (94.1833, 69.9707) ccw construction
  line L1368 (93.2799, 68.1863) -> (80.7714, 74.5195) construction
  arc A85 (79.9395, 77.2982) -> (80.7714, 74.5195) centre (81.6748, 76.3039) ccw construction
  line L1369 (79.9395, 77.2982) -> (84.765, 85.7197) construction
  line L1370 (84.765, 85.7197) -> (84.4494, 85.8991) construction
  line L1371 (84.4494, 85.8991) -> (84.1324, 86.0761) construction
  line L1372 (84.1324, 86.0761) -> (83.8142, 86.2509) construction
  line L1373 (83.8142, 86.2509) -> (83.4947, 86.4233) construction
  line L1374 (83.4947, 86.4233) -> (83.1739, 86.5933) construction
  line L1375 (83.1739, 86.5933) -> (82.8519, 86.7611) construction
  line L1376 (82.8519, 86.7611) -> (82.5287, 86.9264) construction
  line L1377 (82.5287, 86.9264) -> (82.2043, 87.0895) construction
  line L1378 (82.2043, 87.0895) -> (81.8788, 87.2501) construction
  line L1379 (81.8788, 87.2501) -> (81.552, 87.4084) construction
  line L1380 (81.552, 87.4084) -> (81.1818, 87.1685) construction
  line L1381 (81.1818, 87.1685) -> (80.8185, 86.9241) construction
  line L1382 (80.8185, 86.9241) -> (80.4622, 86.6753) construction
  line L1383 (80.4622, 86.6753) -> (80.1132, 86.4222) construction
  line L1384 (80.1132, 86.4222) -> (79.7716, 86.1646) construction
  line L1385 (79.7716, 86.1646) -> (79.4376, 85.9028) construction
  line L1386 (79.4376, 85.9028) -> (79.1113, 85.6366) construction
  line L1387 (79.1113, 85.6366) -> (78.7929, 85.366) construction
  line L1388 (78.7929, 85.366) -> (78.4827, 85.0912) construction
  line L1389 (78.4827, 85.0912) -> (78.181, 84.812) construction
  line L1390 (78.181, 84.812) -> (77.888, 84.5284) construction
  line L1391 (77.888, 84.5284) -> (77.6041, 84.2404) construction
  line L1392 (77.6041, 84.2404) -> (77.3297, 83.9478) construction
  line L1393 (77.3297, 83.9478) -> (77.0654, 83.6507) construction
  line L1394 (77.0654, 83.6507) -> (76.8117, 83.3487) construction
  line L1395 (76.8117, 83.3487) -> (76.5695, 83.0417) construction
  line L1396 (76.5695, 83.0417) -> (76.34, 82.7293) construction
  line L1397 (76.34, 82.7293) -> (76.1248, 82.4108) construction
  line L1398 (76.1248, 82.4108) -> (75.927, 82.0852) construction
  line L1399 (75.927, 82.0852) -> (75.755, 81.7492) construction
  line L1400 (75.755, 81.7492) -> (75.6407, 81.4942) construction
  line L1401 (75.6407, 81.4942) -> (75.519, 81.2516) construction
  line L1402 (75.519, 81.2516) -> (75.3916, 81.0208) construction
  line L1403 (75.3916, 81.0208) -> (75.2614, 80.8008) construction
  line L1404 (75.2614, 80.8008) -> (75.1232, 80.594) construction
  line L1405 (75.1232, 80.594) -> (74.977, 80.4005) construction
  line L1406 (74.977, 80.4005) -> (74.8227, 80.2207) construction
  line L1407 (74.8227, 80.2207) -> (74.666, 80.0524) construction
  line L1408 (74.666, 80.0524) -> (74.5014, 79.8983) construction
  line L1409 (74.5014, 79.8983) -> (74.3269, 79.7593) construction
  line L1410 (74.3269, 79.7593) -> (74.1494, 79.633) construction
  line L1411 (74.1494, 79.633) -> (73.963, 79.5223) construction
  line L1412 (73.963, 79.5223) -> (73.7684, 79.4272) construction
  line L1413 (73.7684, 79.4272) -> (73.5688, 79.3472) construction
  line L1414 (73.5688, 79.3472) -> (73.3575, 79.2855) construction
  line L1415 (73.3575, 79.2855) -> (73.1416, 79.2402) construction
  line L1416 (73.1416, 79.2402) -> (72.9105, 79.2166) construction